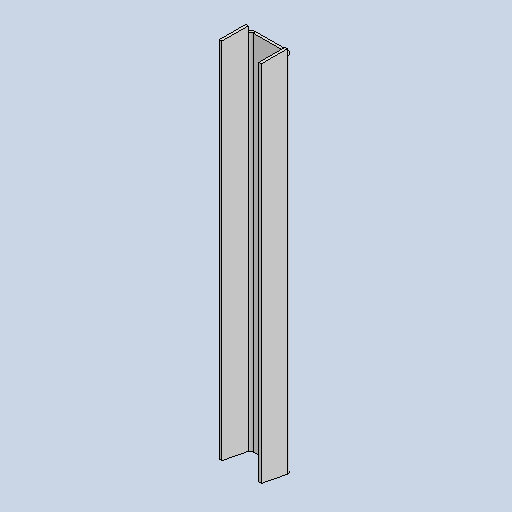
# Autodesk Inventor part: DMF v2.1 gear wheel pin 1
Saved by Autodesk Inventor 2026.2 (Build 302298010, 298A)
## iProperties
Created: 2024-04-30
Part Number: DMF v2.1 gear wheel pin 1
Material: Generic
Document SubType Name: Sheet Metal
Designer: pokla
Stock Number: Барабан_Сектор_Усилителя
Density: 1 g/cm^3
Sheet Metal Rule: Default
Sheet Metal Width: 0,000 mm
Sheet Metal Length: 0,000 mm
Sheet Metal Area: 0,000 mm^2
Appearance: Default
Author: pokla
Autodesk Inventor part; units mm, degrees
ref_plane "YZ Plane" through (0, 0, 0) normal (1, 0, 0) x (0, 1, 0)
ref_plane "XZ Plane" through (0, 0, 0) normal (0, 1, 0) x (-1, 0, 0)
ref_plane "XY Plane" through (0, 0, 0) normal (0, 0, 1) x (1, 0, 0)
sketch "Sketch1" plane through (0, 0, 0) normal (0, 0, 1) x (1, 0, 0)
  line L0 (-16.75, 305) -> (16.75, 305)
  line L1 (16.75, 305) -> (16.75, 0)
  line L2 (16.75, 0) -> (-16.75, 0)
  line L3 (-16.75, 0) -> (-16.75, 305)
  point P0 (0, 0)
  point P1 (0, 0)
  point P2 (0, 0)
  point P3 (0, 0)
  point P4 (0, 0)
  dimension "d27" = 33.5
  dimension "d29" = 305
  measures "d27" distance of L1.end L2.end
  measures "d29" distance of L0.end L1.end
extrude "Plate1" add sketch "Sketch1" against normal blind 2
sketch "Sketch2" plane through (14.75, 305, -2) normal (1, 0, 0) x (0, 1, 0)
  line L0 (-305, 0) -> (0, 0)
  line L1 (0, 0) -> (0, 25)
  line L2 (0, 25) -> (-305, 25)
  line L3 (-305, 25) -> (-305, 0)
  constraints: 6 end point, 1 horizontal, 1 perpendicular, 1 vertical
edge flange "Flange1" height 25 angle 90 thickness 2 bend radius 2 thickness toward (1, 0, 0) relief tear relief width 2 relief depth 1 corner gap 2 corner form 0 edges at (16.75, 152.5, 0) (-16.75, 152.5, 0) wall of the first edge with corners at (14.75, 0, -2) (14.75, 305, -2) (14.75, 305, 23) (14.75, 0, 23)
bend "Bend1"
corner "Corner1"
sketch "Sketch3" plane through (16.75, 0, 23) normal (1, 0, 0) x (0, 0, -1)
  line L0 (0, 305) -> (21, 305)
  line L1 (21, 305) -> (21, 0)
  line L2 (21, 305) -> (21, 310)
  line L3 (21, 310) -> (0, 310)
  line L4 (0, 310) -> (0, 305)
  point P0 (23, 0)
  dimension "d40" = 5
  measures "d40" distance of L0.end L2.end
sheet face with bend "Face2" sketch "Sketch3" thickness 2 toward (-1, 0, 0) bend radius 2
bend "Bend2"
mirror "Mirror1" about plane through (0, 0, 0) normal (1, 0, 0)
sketch "Sketch4" plane through (16.75, 0, 23) normal (1, 0, 0) x (0, 0, -1)
  line L0 (0, 310) -> (0, 0) projected
  line L1 (0, 19.8595) -> (25, 15)
  line L2 (25, 305) -> (25, 0) projected
  line L3 (25, 0) -> (0, 0)
  line L4 (21, 310) -> (0, 310) projected
  point P0 (23, 0)
  dimension "d46" = 295
  dimension "d47" = 11
  constraints: 4 end point, 2 point on line, 1 horizontal
  measures "d46" distance from line of L1.end L4
  measures "d47" angle of L3 L1
extrude "Extrusion1" cut sketch "Sketch4" along normal through all both and the other way through all
equation "\"d47\" = wheel_pin_Angle"
equation "\"d15\" = Thickness"
equation "\"d30\" = BendReliefWidth"
equation "\"d31\" = BendReliefDepth"
equation "\"d32\" = MinimumRemnant"
equation "\"d33\" = TransitionRadius"
equation "\"d34\" = wheel_pin_h"
equation "\"d36\" = BendRadius"
equation "\"d37\" = CornerReliefSize"
equation "\"d38\" = GapSize"
equation "\"d39\" = JacobiRadiusSize"
equation "\"GapSize\" = Thickness"
equation "\"BendRadius\" = Thickness"
equation "\"MinimumRemnant\" = 2 * Thickness"
equation "\"BendReliefDepth\" = 0.5 * Thickness"
equation "\"BendReliefWidth\" = Thickness"
equation "\"CornerReliefSize\" = 4 * Thickness"
equation "\"JacobiRadiusSize\" = BendRadius"
equation "\"TransitionRadius\" = BendRadius"
equation "\"d41\" = BendRadius"
equation "\"d42\" = BendReliefWidth"
equation "\"d44\" = MinimumRemnant"
equation "\"d43\" = BendReliefDepth"
equation "\"d45\" = TransitionRadius"
equation "\"wheel_pin_Angle\" = 11deg"
equation "\"Thickness\" = 2"
equation "\"wheel_pin_h\" = 25"
body "Solid1"
